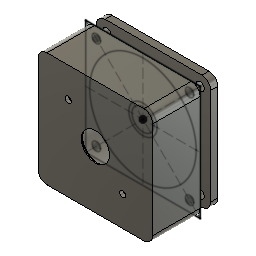
redukce_motoru_simulator_autoskoly (Autodesk Fusion 360 design; units mm, degrees)
Autodesk Fusion 360 part; units mm, degrees
sketch "Sketch1" plane through (0, 0, 0) normal (0, 0, 1) x (1, 0, 0)
  line L0 (-32.5, 32.5) -> (32.5, 32.5)
  line L1 (32.5, 32.5) -> (32.5, -32.5)
  line L2 (32.5, -32.5) -> (-32.5, -32.5)
  line L3 (-32.5, -32.5) -> (-32.5, 32.5)
  line L4 (-32.5, 32.5) -> (32.5, -32.5) construction
  line L5 (32.5, 32.5) -> (-32.5, -32.5) construction
  circle A0 centre (-26.5, 26.5) radius 2.35
  line L6 (-32.5, 0) -> (32.5, 0) construction
  line L7 (0, 32.5) -> (0, -32.5) construction
  circle A1 centre (-26.5, -26.5) radius 2.35
  circle A2 centre (26.5, -26.5) radius 2.35
  circle A3 centre (26.5, 26.5) radius 2.35
  circle A4 centre (0, 0) radius 30.25
  circle A5 centre (0, 0) radius 8
  circle A6 centre (0, 0) radius 6.2
  dimension "d1" = 65
  dimension "d2" = 65
  dimension "d3" = 4.7
  dimension "d4" = 26.5
  dimension "d6" = 360
  dimension "d7" = 60.5
  dimension "d17" = 12.4
  dimension "d18" = 16
  constraint horizontal L0
  constraint perpendicular L0 L1
  constraint parallel L0 L2
  constraint parallel L1 L3
  constraint coincident L4 A4.centre
  constraint coincident L5 A4.centre
  constraint coincident A4.centre A5.centre
  constraint coincident L4 A0.centre
  constraint midpoint L3 L6.start
  constraint midpoint L1 L6.end
  constraint midpoint L0 L7.start
  constraint midpoint L2 L7.end
  constraint concentric A4 A5
  measures "d1" distance of L0.end L1.end
  measures "d2" distance of L0.start L0.end
  measures "d3" diameter of A0
  measures "d4" horizontal distance of A4.centre A0.centre
  measures "d7" diameter of A4
  measures "d17" diameter of A6
  measures "d18" diameter of A5
extrude "Extrude1" add sketch "Sketch1" along normal blind 27 contours L0 L1 L2 L3 makes body 1
sketch "Sketch2" plane through (0, 0, 27) normal (0, 0, 1) x (1, 0, 0)
  circle A0 centre (26.5, -26.5) radius 2.35
  circle A1 centre (-26.5, 26.5) radius 2.35
  circle A2 centre (-26.5, -26.5) radius 2.35
  circle A3 centre (26.5, 26.5) radius 2.35
  circle A4 centre (0, 0) radius 30.25
  line L0 (-32.5, -32.5) -> (32.5, -32.5)
  line L1 (32.5, -32.5) -> (32.5, 32.5)
  line L2 (32.5, 32.5) -> (-32.5, 32.5)
  line L3 (-32.5, 32.5) -> (-32.5, -32.5)
  circle A5 centre (0, 0) radius 8
  line L4 (-32.5, 32.5) -> (32.5, -32.5) construction
  line L5 (32.5, 32.5) -> (-32.5, -32.5) construction
  circle A6 centre (-15.4856, 15.4856) radius 1.75
  circle A7 centre (15.4856, -15.4856) radius 1.75
  dimension "d14" = 16
  dimension "d15" = 3.5
  dimension "d16" = 21.9
  constraint coincident A4.centre A5.centre
  constraint coincident L2.end L3.start
  constraint coincident L0.end L1.start
  constraint coincident L1.end L2.start
  constraint coincident L0.start L3.end
  constraint coincident L4 A6.centre
  constraint symmetric L5 A6 A7
  measures "d14" diameter of A5
  measures "d15" diameter of A6
  measures "d16" distance of A4.centre A6.centre
extrude "Extrude2" add sketch "Sketch2" against normal blind 2 contours A0 | A1 | A2 | A3 | A4 bodies 1
fillet "Fillet1" radius 5 4 edges at (-32.5, 32.5, 13.5) (32.5, 32.5, 13.5) (-32.5, -32.5, 13.5) (32.5, -32.5, 13.5) on bodies 1
extrude "Extrude3" add sketch "Sketch1" along normal blind 14 separate body contours A5 makes body 2
sketch "Sketch3" plane through (0, 0, 14) normal (0, 0, 1) x (1, 0, 0)
  circle A0 centre (0, 0) radius 6.2
  circle A1 centre (0, 0) radius 8
  line L0 (0, 32.5) -> (0, -32.5) construction
  line L1 (0, 0) -> (-0.946, -4.4506) construction
  line L2 (0, 0) -> (0.4286, -4.0775) construction
  line L3 (0.4756, -4.5251) -> (0.4286, -4.0775)
  line L4 (-0.4756, -4.5251) -> (-0.4286, -4.0775)
  arc A2 (-0.4756, -4.5251) -> (0.4756, -4.5251) centre (0, 0) ccw
  line L5 (2.275, -3.9404) -> (2.05, -3.5507)
  arc A3 (1.406, -4.3273) -> (2.275, -3.9404) centre (0, 0) ccw
  line L6 (1.406, -4.3273) -> (1.267, -3.8993)
  line L7 (3.681, -2.6744) -> (3.317, -2.4099)
  arc A4 (3.0445, -3.3813) -> (3.681, -2.6744) centre (0, 0) ccw
  line L8 (3.0445, -3.3813) -> (2.7434, -3.0469)
  line L9 (4.4506, -0.946) -> (4.0104, -0.8524)
  arc A5 (4.1566, -1.8507) -> (4.4506, -0.946) centre (0, 0) ccw
  line L10 (4.1566, -1.8507) -> (3.7455, -1.6676)
  line L11 (4.4506, 0.946) -> (4.0104, 0.8524)
  arc A6 (4.55, 0) -> (4.4506, 0.946) centre (0, 0) ccw
  line L12 (4.55, 0) -> (4.1, 0)
  line L13 (3.681, 2.6744) -> (3.317, 2.4099)
  arc A7 (4.1566, 1.8507) -> (3.681, 2.6744) centre (0, 0) ccw
  line L14 (4.1566, 1.8507) -> (3.7455, 1.6676)
  line L15 (2.275, 3.9404) -> (2.05, 3.5507)
  arc A8 (3.0445, 3.3813) -> (2.275, 3.9404) centre (0, 0) ccw
  line L16 (3.0445, 3.3813) -> (2.7434, 3.0469)
  line L17 (0.4756, 4.5251) -> (0.4286, 4.0775)
  arc A9 (1.406, 4.3273) -> (0.4756, 4.5251) centre (0, 0) ccw
  line L18 (1.406, 4.3273) -> (1.267, 3.8993)
  line L19 (-1.406, 4.3273) -> (-1.267, 3.8993)
  arc A10 (-0.4756, 4.5251) -> (-1.406, 4.3273) centre (0, 0) ccw
  line L20 (-0.4756, 4.5251) -> (-0.4286, 4.0775)
  line L21 (-3.0445, 3.3813) -> (-2.7434, 3.0469)
  arc A11 (-2.275, 3.9404) -> (-3.0445, 3.3813) centre (0, 0) ccw
  line L22 (-2.275, 3.9404) -> (-2.05, 3.5507)
  line L23 (-4.1566, 1.8507) -> (-3.7455, 1.6676)
  arc A12 (-3.681, 2.6744) -> (-4.1566, 1.8507) centre (0, 0) ccw
  line L24 (-3.681, 2.6744) -> (-3.317, 2.4099)
  line L25 (-4.55, 0) -> (-4.1, 0)
  arc A13 (-4.4506, 0.946) -> (-4.55, 0) centre (0, 0) ccw
  line L26 (-4.4506, 0.946) -> (-4.0104, 0.8524)
  line L27 (-4.1566, -1.8507) -> (-3.7455, -1.6676)
  arc A14 (-4.4506, -0.946) -> (-4.1566, -1.8507) centre (0, 0) ccw
  line L28 (-4.4506, -0.946) -> (-4.0104, -0.8524)
  line L29 (-3.0445, -3.3813) -> (-2.7434, -3.0469)
  arc A15 (-3.681, -2.6744) -> (-3.0445, -3.3813) centre (0, 0) ccw
  line L30 (-3.681, -2.6744) -> (-3.317, -2.4099)
  line L31 (-1.406, -4.3273) -> (-1.267, -3.8993)
  arc A16 (-2.275, -3.9404) -> (-1.406, -4.3273) centre (0, 0) ccw
  line L32 (-2.275, -3.9404) -> (-2.05, -3.5507)
  arc A17 (-1.267, -3.8993) -> (-0.4286, -4.0775) centre (0, 0) ccw
  arc A18 (-2.7434, -3.0469) -> (-2.05, -3.5507) centre (0, 0) ccw
  arc A19 (-3.7455, -1.6676) -> (-3.317, -2.4099) centre (0, 0) ccw
  arc A20 (-4.1, 0) -> (-4.0104, -0.8524) centre (0, 0) ccw
  arc A21 (-3.7455, 1.6676) -> (-4.0104, 0.8524) centre (0, 0) ccw
  arc A22 (-2.7434, 3.0469) -> (-3.317, 2.4099) centre (0, 0) ccw
  arc A23 (-1.267, 3.8993) -> (-2.05, 3.5507) centre (0, 0) ccw
  arc A24 (0.4286, 4.0775) -> (-0.4286, 4.0775) centre (0, 0) ccw
  arc A25 (2.05, 3.5507) -> (1.267, 3.8993) centre (0, 0) ccw
  arc A26 (4.0104, -0.8524) -> (4.1, 0) centre (0, 0) ccw
  arc A27 (3.317, -2.4099) -> (3.7455, -1.6676) centre (0, 0) ccw
  arc A28 (0.4286, -4.0775) -> (1.267, -3.8993) centre (0, 0) ccw
  arc A29 (2.05, -3.5507) -> (2.7434, -3.0469) centre (0, 0) ccw
  arc A30 (4.0104, 0.8524) -> (3.7455, 1.6676) centre (0, 0) ccw
  arc A31 (3.317, 2.4099) -> (2.7434, 3.0469) centre (0, 0) ccw
  dimension "d21" = 9.1
  dimension "d23" = 8.2
  dimension "d24" = 6
  dimension "d26" = 360
  constraint coincident A0.centre A1.centre
  constraint symmetric L0 L3.start L4.start
  constraint symmetric L0 L2.end L4.end
  constraint concentric A17 A28
  constraint concentric A18 A28
  constraint concentric A19 A28
  constraint concentric A20 A28
  constraint concentric A21 A28
  constraint concentric A22 A28
  constraint concentric A23 A28
  constraint concentric A24 A28
  constraint concentric A25 A28
  constraint concentric A28 A30
  constraint concentric A26 A28
  constraint concentric A27 A28
  constraint concentric A28 A29
  constraint coincident L13.end A30
  constraint concentric A30 A31
  measures "d21" diameter of A2
  measures "d23" diameter of A28
  measures "d24" angle of L0 L2
extrude "Extrude4" add sketch "Sketch3" against normal blind 5 contours A0 bodies 2
chamfer "Chamfer1" distance 1.5 angle 45 1 edges at (-7.4586, -2.8929, 25) on bodies 1
extrude "Extrude5" add sketch "Sketch1" along normal blind 4 from surface at -10 separate body contours L0 L1 L2 L3 | A4 | A5 | A6 makes body 3
fillet "Fillet2" radius 5 4 edges at (-32.5, 32.5, -8) (-32.5, -32.5, -8) (32.5, 32.5, -8) (32.5, -32.5, -8) on bodies 3
hidden bodies 2
equation "d2 = d1"
equation "d4 = ( 53 / 2 ) * 1 mm"
equation "d16 = ( ( 46.3 - 2.5 ) / 2 ) * 1 mm"
named bodies: "stepper motor mount", "axis connect", "position sensor cover"
